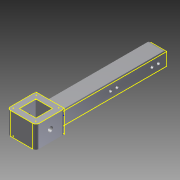
# Autodesk Inventor part: proteccionQuadCopter3_B
Saved by Autodesk Inventor 2012 (Build 160160000, 160)
## iProperties
Created: 2013-01-12
Part Number: proteccionQuadCopter3_B
Material: Default
Document SubType Name: Modeling
Designer: Pablo
Density: 1 g/cm^3
Author: Pablo
Autodesk Inventor part; units mm, degrees
ref_plane "YZ Plane" through (0, 0, 0) normal (1, 0, 0) x (0, 1, 0)
ref_plane "XZ Plane" through (0, 0, 0) normal (0, 1, 0) x (-1, 0, 0)
ref_plane "XY Plane" through (0, 0, 0) normal (0, 0, 1) x (1, 0, 0)
sketch "Boceto1" plane through (0, 0, 0) normal (0, 0, 1) x (1, 0, 0)
  line L0 (0, 0) -> (10, 0)
  line L1 (10, 0) -> (10, -10)
  line L2 (10, -10) -> (0, -10)
  line L3 (0, -10) -> (0, 0)
  line L4 (0, 0) -> (0, 4)
  line L5 (0, 4) -> (-4, 4)
  line L6 (-4, 4) -> (-4, -14)
  line L7 (-4, -14) -> (14, -14)
  line L8 (14, -14) -> (14, 4)
  line L9 (14, 4) -> (10, 4)
  line L10 (10, 4) -> (10, 40)
  line L11 (10, 40) -> (0, 40)
  line L12 (0, 40) -> (0, 4)
  line L13 (10, 40) -> (10, 42)
  line L14 (10, 42) -> (0, 42)
  line L15 (0, 42) -> (0, 40)
  line L16 (10, 42) -> (10, 66)
  line L17 (10, 66) -> (0, 66)
  line L18 (0, 66) -> (0, 42)
  line L19 (10, 66) -> (10, 68)
  line L20 (10, 68) -> (0, 68)
  line L21 (0, 68) -> (0, 66)
  line L22 (0, 68) -> (0, 72)
  line L23 (0, 72) -> (10, 72)
  line L24 (10, 72) -> (10, 68)
  dimension "d0" = 10
  dimension "d1" = 10
  dimension "d2" = 4
  dimension "d3" = 4
  dimension "d4" = 18
  dimension "d5" = 18
  dimension "d6" = 18
  dimension "d7" = 36
  dimension "d8" = 10
  dimension "d9" = 2
  dimension "d10" = 24
  dimension "d11" = 10
  dimension "d12" = 2
  dimension "d13" = 10
  dimension "d14" = 4
  dimension "d15" = 10
  dimension "d16" = 4
  constraints: 50 end point, 10 parallel, 8 perpendicular, 3 collinear, 1 horizontal
  measures "d0" distance of L0.start L0.end
  measures "d1" distance of L0.end L1.end
  measures "d2" distance of L0.start L4.end
  measures "d3" distance of L4.end L5.end
  measures "d4" distance of L5.end L6.end
  measures "d5" distance of L6.end L7.end
  measures "d6" distance of L7.end L8.end
  measures "d7" distance of L9.end L10.end
  measures "d8" distance of L10.end L11.end
  measures "d9" distance of L10.end L13.end
  measures "d10" distance of L13.end L16.end
  measures "d11" distance of L16.end L17.end
  measures "d12" distance of L16.end L19.end
  measures "d13" distance of L19.end L20.end
  measures "d14" distance of L20.end L22.end
  measures "d15" distance of L22.end L23.end
  measures "d16" distance of L23.end L19.end
extrude "Extrusión1" add sketch "Boceto1" along normal blind 8
sketch "Boceto2" plane through (10, 4, 0) normal (1, 0, 0) x (0, 0, -1)
  line L0 (-8, 68) -> (-8, 0) projected
  line L1 (0, 0) -> (-8, 0) projected
  line L2 (0, 0) -> (0, 68) projected
  line L3 (0, 68) -> (-8, 68) projected
  point P0 (0, -4)
sketch "Boceto3" plane through (0, 72, 0) normal (0, 1, 0) x (1, 0, 0)
  line L0 (0, -8) -> (10, -8) projected
  line L1 (10, 0) -> (10, -8) projected
  line L2 (10, 0) -> (0, 0) projected
  line L3 (0, 0) -> (0, -8) projected
sketch "Boceto4" plane through (10, 4, 0) normal (1, 0, 0) x (0, 0, -1)
  line L0 (0, 0) -> (0, 68) projected
  line L1 (0, 68) -> (0, 63)
  line L2 (0, 63) -> (-4, 63)
  line L3 (-4, 63) -> (-4, 37)
  circle A0 centre (-4, 63) radius 1
  circle A1 centre (-4, 37) radius 1
  point P0 (0, -4)
  dimension "d19" = 5
  dimension "d20" = 26
  dimension "d21" = 2
  dimension "d22" = 2
  constraints: 6 end point, 2 centre point, 2 coincident, 1 parallel, 1 perpendicular, 1 point on line
  measures "d19" distance of L0.end L1.end
  measures "d20" distance of L2.end L3.end
  measures "d21" diameter of A0
  measures "d22" diameter of A1
extrude "Extrusión2" cut sketch "Boceto4" against normal up to surface (10 mm away)
sketch "Boceto5" plane through (-4, -14, 0) normal (0, -1, 0) x (1, 0, 0)
  line L0 (0, 8) -> (18, 0)
  point P0 (4, 0)
  constraints: 2 end point
extrude "Extrusión3" [suppressed]
sketch "Boceto6" plane through (0, 0, 0) normal (0, 0, -1) x (-1, 0, 0)
  line L0 (-10, 0) -> (0, 0) projected
  line L1 (0, 0) -> (0, -10) projected
  line L2 (0, -10) -> (-10, -10) projected
  line L3 (-10, -10) -> (-10, 0) projected
  line L4 (0, 72) -> (0, 4) projected
  line L5 (-10, 72) -> (0, 72) projected
  line L6 (-10, 4) -> (-10, 72) projected
  line L7 (-14, 4) -> (-10, 4) projected
  line L8 (-14, -14) -> (-14, 4) projected
  line L9 (4, -14) -> (-14, -14) projected
  line L10 (4, 4) -> (4, -14) projected
  line L11 (0, 4) -> (4, 4) projected
extrude "Extrusión4" add sketch "Boceto6" along normal blind 1
sketch "Boceto7" plane through (0, 0, 8) normal (0, 0, 1) x (1, 0, 0)
  line L0 (0, 0) -> (10, 0) projected
  line L1 (10, 0) -> (10, -10) projected
  line L2 (10, -10) -> (0, -10) projected
  line L3 (0, -10) -> (0, 0) projected
  line L4 (0, 4) -> (0, 72) projected
  line L5 (-4, 4) -> (0, 4) projected
  line L6 (-4, -14) -> (-4, 4) projected
  line L7 (14, -14) -> (-4, -14) projected
  line L8 (14, 4) -> (14, -14) projected
  line L9 (10, 4) -> (14, 4) projected
  line L10 (10, 72) -> (10, 4) projected
  line L11 (0, 72) -> (10, 72) projected
extrude "Extrusión5" add sketch "Boceto7" along normal blind 1
sketch "Boceto8" plane through (0, 0, 9) normal (0, 0, 1) x (1, 0, 0)
  line L0 (10, 0) -> (10, -10) projected
  line L1 (10, -10) -> (0, -10) projected
  line L2 (0, 0) -> (10, 0) projected
  line L3 (-4, 4) -> (0, 4) projected
  line L4 (10, 4) -> (14, 4) projected
  line L5 (10, 72) -> (10, 4) projected
  line L6 (0, 4) -> (10, 4)
  line L7 (-4, 4) -> (0, 4)
  line L8 (-4, 4) -> (-4, -14)
  line L9 (14, -14) -> (-4, -14)
  line L10 (14, -14) -> (14, 4)
  line L11 (10, 4) -> (14, 4)
  line L12 (0, 0) -> (10, 0)
  line L13 (10, 0) -> (10, -10)
  line L14 (10, -10) -> (0, -10)
  line L15 (0, -10) -> (0, 0)
  constraints: 20 end point, 5 collinear, 5 perpendicular
extrude "Extrusión6" add sketch "Boceto8" along normal blind 4
sketch "Boceto9" plane through (10, 4, -1) normal (0, 1, 0) x (1, 0, 0)
  line L0 (4, 0) -> (4, -14) projected
  line L1 (4, 0) -> (0, 0) projected
  line L2 (0, 0) -> (0, -10) projected
  line L3 (-10, -10) -> (0, -10) projected
  line L4 (-10, -10) -> (-10, 0) projected
  line L5 (-10, 0) -> (-14, 0) projected
  line L6 (-14, 0) -> (-14, -14) projected
  line L7 (-14, -14) -> (4, -14) projected
  line L8 (0, -10) -> (4, -10)
  line L9 (-10, -10) -> (-14, -10)
  point P0 (-10, -1)
  constraints: 4 end point, 2 perpendicular, 2 point on line
fillet "Empalme1" radius 4 2 edges at (10, 4, 4) (0, 4, 4)
chamfer "Chaflán1" distance 4 angle 45 3 edges at (11.9999, 4, 9) (5, 4, 9) (-1.9999, 4, 9)
fillet "Empalme2" radius 2 11 edges at (14, -14, 6) (-4, -14, 6) (13.9999, 4, 11) (14, 4, 6) (13.9999, 4, 4) (14, 4, -1) (-3.9999, 4, 11) (-3.9999, 4, 4) (-3.9999, 4, -1) (-4, 4, 6) (5, 72, 9)
sketch "Boceto10" plane through (0, 0, 13) normal (0, 0, 1) x (1, 0, 0)
  line L0 (10, 0) -> (10, -10) projected
  line L1 (10, -10) -> (0, -10) projected
  line L2 (0, -10) -> (0, 0) projected
  line L3 (0, 0) -> (10, 0) projected
  line L4 (-4, -12) -> (-4, 2.3431) projected
  line L5 (0, 0) -> (-0.2, 0)
  line L6 (-0.2, 0) -> (-0.2, -10.2)
  line L7 (-0.2, -10.2) -> (10.2, -10.2)
  line L8 (10.2, -10.2) -> (10.2, 0.2)
  line L9 (10.2, 0.2) -> (-0.2, 0.2)
  line L10 (-0.2, 0.2) -> (-0.2, 0)
  dimension "d39" = 0.2
  dimension "d40" = 10.2
  dimension "d41" = 10.4
  dimension "d42" = 10.4
  dimension "d43" = 10.4
  constraints: 12 end point, 3 perpendicular, 2 parallel
  measures "d39" distance of L2.end L5.end
  measures "d40" distance of L5.end L6.end
  measures "d41" distance of L6.end L7.end
  measures "d42" distance of L7.end L8.end
  measures "d43" distance of L8.end L9.end
extrude "Extrusión7" cut sketch "Boceto10" against normal blind 20
sketch "Boceto11" plane through (0, 0, 13) normal (0, 0, 1) x (1, 0, 0)
  line L0 (10.2, -10.2) -> (-0.2, -10.2) projected
  line L1 (-0.2, -10.2) -> (-0.2, 0.2) projected
  line L2 (-0.2, 0.2) -> (10.2, 0.2) projected
  line L3 (10.2, 0.2) -> (10.2, -10.2) projected
  arc A0 (-3.1202, 4) -> (-4, 2.3431) centre (-2, 2.3431) ccw projected
  line L4 (-4, -12) -> (-4, 2.3431) projected
  arc A1 (-4, -12) -> (-2, -14) centre (-2, -12) ccw projected
  line L5 (12, -14) -> (-2, -14) projected
  arc A2 (12, -14) -> (14, -12) centre (12, -12) ccw projected
  line L6 (14, 2.3431) -> (14, -12) projected
  arc A3 (14, 2.3431) -> (13.1202, 4) centre (12, 2.3431) ccw projected
  line L7 (-3.1202, 4) -> (13.1202, 4) projected
  point P0 (0, 0)
sketch "Boceto12" plane through (-2, -14, -1) normal (0, -1, 0) x (1, 0, 0)
  line L0 (0, 0) -> (0, 14) projected
  line L1 (0, 0) -> (14, 0) projected
  line L2 (14, 14) -> (14, 0) projected
  line L3 (14, 14) -> (0, 14) projected
  point P0 (2, 1)
sketch "Boceto13" plane through (-2, -14, -1) normal (0, -1, 0) x (1, 0, 0)
  line L0 (0, 0) -> (0, 14) projected
  line L1 (0, 0) -> (14, 0) projected
  line L2 (14, 14) -> (14, 0) projected
  line L3 (14, 14) -> (0, 14) projected
  point P0 (2, 1)
sketch "Boceto14" plane through (14, -12, 13) normal (1, 0, 0) x (0, 0, -1)
  circle A0 centre (7, 7.1716) radius 1.6
  point P0 (13, 12)
  dimension "d46" = 3.2
  constraints: 1 centre point
  measures "d46" diameter of A0
extrude "Extrusión8" cut sketch "Boceto14" along normal mid plane 40
sketch "Boceto15" plane through (10, 8, -1) normal (1, 0, 0) x (0, 0, -1)
  circle A0 centre (-5, 55) radius 1
  circle A1 centre (-5, 29) radius 1
  constraints: 2 centre point
extrude "Extrusión9" cut sketch "Boceto15" against normal up to surface (10 mm away)
